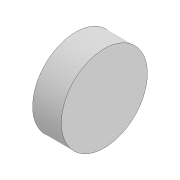
# Autodesk Inventor part: wheel
Saved by Autodesk Inventor 2022 (Build 260153000, 153)
## iProperties
Created: 2024-03-20
Part Number: wheel
Material: Generic
Document SubType Name: Modeling
Designer: david
Density: 1 g/cm^3
Appearance: Default
Author: david
Autodesk Inventor part; units mm, degrees
ref_plane "YZ Plane" through (0, 0, 0) normal (1, 0, 0) x (0, 1, 0)
ref_plane "XZ Plane" through (0, 0, 0) normal (0, 1, 0) x (-1, 0, 0)
ref_plane "XY Plane" through (0, 0, 0) normal (0, 0, 1) x (1, 0, 0)
sketch "Sketch1" plane through (0, 0, 0) normal (1, 0, 0) x (0, 1, 0)
  circle A0 centre (0, 0) radius 30
  dimension "diameter" = 60
  constraints: 1 centre point, 1 coincident
  measures "diameter" diameter of A0
extrude "Extrusion1" add sketch "Sketch1" along normal blind 20
sketch "Sketch2" plane through (0, 0, 0) normal (-1, 0, 0) x (0, 0, 1)
  line L0 (-2, -2.2361) -> (2, -2.2361) construction
  line L1 (2, -2.2361) -> (2, 2.2361)
  line L2 (2, 2.2361) -> (-2, 2.2361) construction
  line L3 (-2, 2.2361) -> (-2, -2.2361)
  line L4 (-2, -2.2361) -> (2, 2.2361) construction
  line L5 (2, -2.2361) -> (0, 0) construction
  arc A0 (-2, -2.2361) -> (2, -2.2361) centre (0, 0) ccw
  arc A1 (-2, 2.2361) -> (-2, -2.2361) centre (0, 0) ccw construction
  arc A2 (2, 2.2361) -> (-2, 2.2361) centre (0, 0) ccw
  arc A3 (2, -2.2361) -> (2, 2.2361) centre (0, 0) ccw construction
  line L6 (0, 0) -> (-2, 2.2361) construction
  dimension "d5" = 4
  dimension "d7" = 6
  constraints: 14 end point, 8 point on circle, 4 centre point, 2 parallel, 1 coincident, 1 horizontal, 1 midpoint, 1 perpendicular
  measures "d5" distance of L1.end L2.end
  measures "d7" diameter of A2
extrude "Extrusion2" cut sketch "Sketch2" against normal blind 7
body "Solid1"
